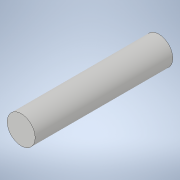
# Autodesk Inventor part: Hydraulic tank
Saved by Autodesk Inventor 2021 (Build 250183000, 183)
## iProperties
Created: 2020-10-20
Part Number: Hydraulic tank
Material: Generic
Document SubType Name: Modeling
Designer: Jawal
Density: 1 g/cm^3
Appearance: Default
Mass: 7547.19 g
Surface Area: 2660.54 cm^2
Volume: 7547.19 cm^3
Author: Jawal
Autodesk Inventor part; units mm, degrees
ref_plane "YZ Plane" through (0, 0, 0) normal (1, 0, 0) x (0, 1, 0)
ref_plane "XZ Plane" through (0, 0, 0) normal (0, 1, 0) x (-1, 0, 0)
ref_plane "XY Plane" through (0, 0, 0) normal (0, 0, 1) x (1, 0, 0)
sketch "Sketch1" plane through (0, 0, 0) normal (0, 0, 1) x (1, 0, 0)
  circle A0 centre (0, 0) radius 62.5
  dimension "d2" = 615
  dimension "d4" = 125
  constraints: 1 centre point
  measures "d4" diameter of A0
extrude "Extrusion1" add sketch "Sketch1" along normal blind 615
body "Solid1"
